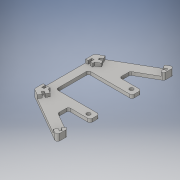
# Autodesk Inventor part: walle
Saved by Autodesk Inventor 2016 SP2 (Build 200236200, 236)
## iProperties
Created: 2016-10-31
Part Number: walle
Material: Generic
Document SubType Name: Modeling
Designer: xwang797
Density: 1 g/cm^3
Appearance: Default
Author: xwang797
Autodesk Inventor part; units mm, degrees
ref_plane "YZ Plane" through (0, 0, 0) normal (1, 0, 0) x (0, 1, 0)
ref_plane "XZ Plane" through (0, 0, 0) normal (0, 1, 0) x (-1, 0, 0)
ref_plane "XY Plane" through (0, 0, 0) normal (0, 0, 1) x (1, 0, 0)
sketch "Sketch1" plane through (0, 0, 0) normal (0, 1, 0) x (-1, 0, 0)
  line L0 (0, -15) -> (40, -15)
  line L1 (0, -54.7509) -> (0, -44.7509)
  line L2 (20, -23.5) -> (0, -23.5)
  line L3 (0, -23.5) -> (0, -15)
  circle A0 centre (5.2574, -19.75) radius 1.75
  line L4 (47.2, -27.5) -> (0, -54.7509)
  line L5 (0, -44.7509) -> (20, -33.2039)
  line L6 (20, -23.5) -> (20, -33.2039)
  line L7 (0, 15) -> (40, 15)
  line L8 (0, 54.7509) -> (0, 44.7509)
  line L9 (20, 23.5) -> (0, 23.5)
  line L10 (0, 23.5) -> (0, 15)
  circle A1 centre (5.2574, 19.75) radius 1.75
  line L11 (47.2, 27.5) -> (0, 54.7509)
  line L12 (0, 44.7509) -> (20, 33.2039)
  line L13 (20, 23.5) -> (20, 33.2039)
  line L14 (47.2, 27.5) -> (47.2, -27.5)
  line L15 (40, 15) -> (40, -15)
  line L16 (56.64, 0) -> (-9.44, 0) projected
  line L17 (0, -76.6513) -> (0, 76.6513) projected
  point P0 (0, 0)
  point P1 (0, 19.25)
  dimension "d3" = 15
  dimension "d6" = 5.2573
  dimension "d7" = 3.5
  dimension "d8" = 8.5
  dimension "d10" = 10
  dimension "d13" = 47.2
  dimension "d15" = 39.5
  dimension "d29" = 15
  dimension "d30" = 5.2573
  dimension "d31" = 40
  dimension "d32" = 19.75
  dimension "d33" = 8.5
  dimension "d34" = 20
  dimension "d35" = 20
  dimension "d37" = 60
  dimension "d38" = 60
  dimension "d39" = 55
  dimension "d40" = 27.5
  dimension "d41" = 10
  dimension "d68" = 21.2509
  constraints: 32 end point, 8 vertical, 3 horizontal, 2 centre point, 2 collinear, 2 parallel, 2 point on line, 1 equal radius, 1 midpoint, 1 perpendicular
  measures "d3" distance of point (0, 0) L0.start
  measures "d6" distance from line of L3 A0.centre
  measures "d7" diameter of A0
  measures "d8" distance of L2.end L0.start
  measures "d10" distance of L1.start L1.end
  measures "d13" horizontal distance of L4.start L1.start
  measures "d15" distance of A0.centre A1.centre
  measures "d29" distance from line of point (0, 0) L7
  measures "d30" horizontal distance of point (0, 0) A1.centre
  measures "d31" distance between parallel lines of L17 L15
  measures "d32" distance from line of L16 A0.centre
  measures "d33" distance between parallel lines of L7 L9
  measures "d34" distance of L2.start L2.end
  measures "d35" distance of L9.start L9.end
  measures "d37" angle of L4 L14
  measures "d38" angle of L11 L14
  measures "d39" distance of L11.start L4.start
  measures "d40" distance from line of L16 L4.start
  measures "d41" distance of L8.start L8.end
  measures "d68" distance from line of L8.end L9
extrude "Extrusion1" add sketch "Sketch1" along normal blind 3 contours L0 L15 L16 L14 L4 L1 L5 L6 L2 L3 | L15 L7 L10 L9 L13 L12 L8 L11 L14 L16
sketch "Sketch2" plane through (0, 3, 0) normal (0, 1, 0) x (1, 0, 0)
  line L0 (-42.8964, 23) -> (-44.8964, 23)
  line L1 (-2.0164, 49.7415) -> (-1.0164, 48.0094)
  line L2 (-40.8535, 25.0094) -> (-41.8535, 26.7415)
  line L3 (-1.0164, -48.0094) -> (-2.0164, -49.7415)
  line L4 (-41.8535, -26.7415) -> (-40.8535, -25.0094)
  line L5 (-40.9205, -31.1255) -> (-39.2554, -28.2415)
  line L6 (-38.2554, -26.5094) -> (-36.5904, -23.6255)
  line L7 (-42.8964, -19.564) -> (-40.5928, -19.564)
  line L8 (-44.8964, -19.564) -> (-47.2, -19.564)
  line L9 (-47.2, 27.5) -> (-47.2, -27.5) projected
  line L10 (-47.2, -27.5) -> (-40.9205, -31.1255)
  line L11 (-47.2, -27.5) -> (0, -54.7509) projected
  line L12 (-4.6144, -48.2415) -> (-6.2795, -51.1255)
  line L13 (-3.6144, -46.5094) -> (-1.9494, -43.6255)
  line L14 (0, -44.7509) -> (-20, -33.2039) projected
  line L15 (-39.2554, 28.2415) -> (-40.9205, 31.1255)
  line L16 (-38.2554, 26.5094) -> (-36.5904, 23.6255)
  line L17 (-3.6144, 46.5094) -> (-1.9494, 43.6255)
  line L18 (-4.6144, 48.2415) -> (-6.2795, 51.1255)
  line L19 (-38.2554, -26.5094) -> (-40.8535, -25.0094)
  line L20 (-41.8535, -26.7415) -> (-39.2554, -28.2415)
  line L21 (-42.8964, -23) -> (-42.8964, -19.564)
  line L22 (-4.6144, -48.2415) -> (-2.0164, -49.7415)
  line L23 (-3.6144, -46.5094) -> (-1.0164, -48.0094)
  line L24 (-6.2795, -51.1255) -> (0, -54.7509)
  line L25 (0, -54.7509) -> (0, -44.7509)
  line L26 (0, -44.7509) -> (-1.9494, -43.6255)
  line L27 (-40.8535, 25.0094) -> (-38.2554, 26.5094)
  line L28 (-41.8535, 26.7415) -> (-39.2554, 28.2415)
  line L29 (-3.6144, 46.5094) -> (-1.0164, 48.0094)
  line L30 (-4.6144, 48.2415) -> (-2.0164, 49.7415)
  line L31 (-1.9494, 43.6255) -> (0, 44.7509)
  line L32 (0, 54.7509) -> (-6.2795, 51.1255)
  line L33 (0, 44.7509) -> (0, 54.7509)
  line L34 (-42.8964, 23) -> (-42.8964, 19.564)
  line L35 (-42.8964, 19.564) -> (-40.5928, 19.564)
  line L36 (-44.8964, 19.564) -> (-47.2, 19.564)
  line L37 (-47.2, 19.564) -> (-47.2, 27.5)
  line L38 (-47.2, 27.5) -> (-40.9205, 31.1255)
  line L39 (0, 54.7509) -> (-47.2, 27.5) projected
  line L40 (-20, 33.2039) -> (0, 44.7509) projected
  line L41 (-44.8964, -19.564) -> (-44.8964, -23)
  line L42 (-44.8964, -23) -> (-42.8964, -23)
  line L43 (-36.5904, 23.6255) -> (-40.5928, 21.3147)
  line L44 (-36.5904, -23.6255) -> (-40.5928, -21.3147)
  line L45 (-40.5928, -21.3147) -> (-40.5928, -19.564)
  line L46 (-40.5928, 19.564) -> (-40.5928, 21.3147)
  line L47 (-47.2, -27.5) -> (-47.2, -19.564)
  line L48 (-44.8964, 19.564) -> (-44.8964, 23)
  point P0 (0, 0)
  dimension "d20" = 2
  dimension "d21" = 46
  dimension "d25" = 2
  dimension "d44" = 3.3301
  dimension "d45" = 3.3301
  dimension "d46" = 46
  dimension "d47" = 3
  dimension "d48" = 3
  dimension "d49" = 7.2509
  dimension "d50" = 7.2509
  dimension "d53" = 3.3301
  dimension "d54" = 3.3301
  dimension "d55" = 3
  dimension "d56" = 3
  dimension "d57" = 7.2509
  dimension "d58" = 7.2509
  dimension "d59" = 2
  dimension "d61" = 2.3036
  dimension "d62" = 2.3036
  dimension "d63" = 2.3036
  dimension "d64" = 2.3036
  dimension "d72" = 46
  dimension "d73" = 2
  dimension "d74" = 2
  dimension "d75" = 3.3301
  dimension "d76" = 3.3301
  dimension "d77" = 7.936
  dimension "d78" = 7.936
  constraints: 88 end point, 18 collinear, 15 parallel, 10 perpendicular, 7 equal length, 4 point on line, 4 vertical, 1 horizontal
  measures "d20" distance of L1.start L1.end
  measures "d21" distance of L2.end L1.start
  measures "d25" distance of L3.start L3.end
  measures "d44" distance between parallel lines of L23 L14
  measures "d45" distance between parallel lines of L22 L11
  measures "d46" distance between parallel lines of L4 L3
  measures "d47" distance between parallel lines of L3 L13
  measures "d48" distance between parallel lines of L6 L4
  measures "d49" distance from line of L11.end L12
  measures "d50" distance from line of L9.end L5
  measures "d53" distance between parallel lines of L39 L30
  measures "d54" distance between parallel lines of L29 L40
  measures "d55" distance between parallel lines of L18 L1
  measures "d56" distance between parallel lines of L15 L2
  measures "d57" distance from line of L32.start L18
  measures "d58" distance from line of L9.start L15
  measures "d59" distance of L0.start L0.end
  measures "d61" distance of L34.end L35.end
  measures "d62" distance of L36.start L36.end
  measures "d63" distance of L7.start L7.end
  measures "d64" distance of L8.start L8.end
  measures "d72" distance of L0.end L41.end
  measures "d73" distance of L41.end L21.start
  measures "d74" distance from line of L4.start L19
  measures "d75" distance from line of L5.end L11
  measures "d76" distance from line of L6.start L44
  measures "d77" distance of L36.end L9.start
  measures "d78" distance of L8.end L9.end
extrude "Extrusion2" add sketch "Sketch2" along normal blind 3
fillet "Fillet1" radius 2 16 edges at (-47.2, 3, -27.5) (-47.2, 3, 27.5) (0, 3, 54.7509) (0, 3, 44.7509) (0, 1.5, -15) (0, 1.5, 23.5) (0, 1.5, 15) (0, 1.5, -23.5) (0, 3, -44.7509) (0, 3, -54.7509) (-20, 1.5, -23.5) (-20, 1.5, -33.2039) (-20, 1.5, 33.2039) (-20, 1.5, 23.5) (-40, 1.5, 15) (-40, 1.5, -15)
equation "\"d30\" = d6"
equation "\"d32\" = 0.5 * d15"
equation "\"d33\" = d8"
equation "\"d35\" = d34"
body "Solid1"
